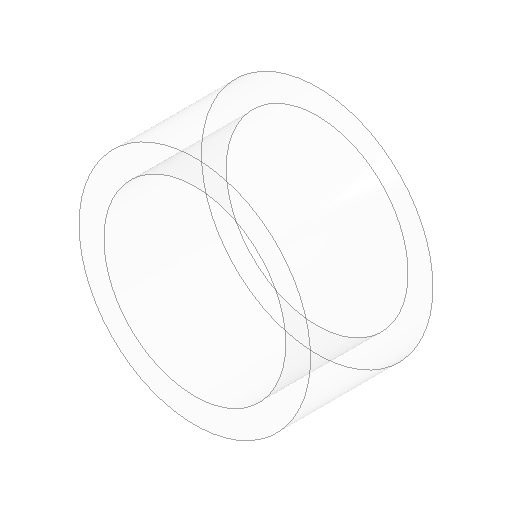
# Autodesk Inventor part: Separador
Saved by Autodesk Inventor 2025.3 (Build 293356000, 356)
## iProperties
Created: 2025-11-11
Part Number: Separador
Material: PMMA Plastic
Document SubType Name: Modeling
Designer: Gabriel Bojaca
Density: 1.188 g/cm^3
Appearance: Polycarbonate - Clear
Author: Gabriel Bojaca
Autodesk Inventor part; units mm, degrees
ref_plane "YZ Plane" through (0, 0, 0) normal (1, 0, 0) x (0, 1, 0)
ref_plane "XZ Plane" through (0, 0, 0) normal (0, 1, 0) x (-1, 0, 0)
ref_plane "XY Plane" through (0, 0, 0) normal (0, 0, 1) x (1, 0, 0)
sketch "Sketch1" plane through (0, 0, 0) normal (0, 0, 1) x (1, 0, 0)
  circle A0 centre (0, 0) radius 3.5
  circle A1 centre (0, 0) radius 1.5
  dimension "d0" = 7
  dimension "d1" = 3
  constraints: 2 centre point, 2 coincident
  measures "d0" diameter of A0
  measures "d1" diameter of A1
extrude "Extrusion1" add sketch "Sketch1" along normal blind 3.7
sketch "Sketch2" plane through (0, 0, 3.7) normal (0, 0, 1) x (1, 0, 0)
  point P0 (0, 0)
hole "Hole1" at (0, 0, 3.7) direction (0, 0, -1) diameter 5.5 end through all
body "Solid1"
